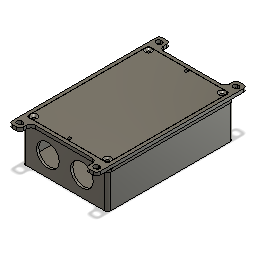
box (Autodesk Fusion 360 design; units mm, degrees)
Autodesk Fusion 360 part; units mm, degrees
sketch "Sketch1" plane through (0, 0, 0) normal (0, 1, 0) x (1, 0, 0)
  line L0 (-39, 48.75) -> (39, 48.75)
  line L1 (39, 48.75) -> (39, -66.25)
  line L2 (39, -66.25) -> (-39, -66.25)
  line L3 (-39, -66.25) -> (-39, 48.75)
  line L4 (0, 70.8126) -> (0, -70.8126) construction
  line L5 (-33.9373, 0) -> (33.9373, 0) construction
  line L6 (-32.25, 35.75) -> (32.25, 35.75) construction
  line L7 (32.25, 35.75) -> (32.25, -35.75) construction
  line L8 (32.25, -35.75) -> (-32.25, -35.75) construction
  line L9 (-32.25, -35.75) -> (-32.25, 35.75) construction
  line L10 (-37, 46.75) -> (37, 46.75)
  line L11 (37, 46.75) -> (37, -64.25)
  line L12 (37, -64.25) -> (-37, -64.25)
  line L13 (-37, -64.25) -> (-37, 46.75)
  circle A0 centre (-32.25, -35.75) radius 3
  circle A1 centre (32.25, -35.75) radius 3
  circle A2 centre (32.25, 35.75) radius 3
  circle A3 centre (-32.25, 35.75) radius 3
  line L14 (-31, 46.75) -> (-31, 43.35)
  line L15 (-33.6, 40.75) -> (-37, 40.75)
  circle A4 centre (-33.6, 43.35) radius 1.3
  arc A5 (-33.6, 40.75) -> (-31, 43.35) centre (-33.6, 43.35) ccw
  line L16 (-33.6, 43.35) -> (-31, 43.35) construction
  line L17 (-33.6, 43.35) -> (-33.6, 40.75) construction
  line L18 (33.6, 40.75) -> (37, 40.75)
  arc A6 (31, 43.35) -> (33.6, 40.75) centre (33.6, 43.35) ccw
  circle A7 centre (33.6, 43.35) radius 1.3
  line L19 (31, 46.75) -> (31, 43.35)
  line L20 (-31, -60.85) -> (-31, -64.25)
  arc A8 (-31, -60.85) -> (-33.6, -58.25) centre (-33.6, -60.85) ccw
  line L21 (-37, -58.25) -> (-33.6, -58.25)
  circle A9 centre (-33.6, -60.85) radius 1.3
  line L22 (-33.6, -60.85) -> (-33.6, -58.25) construction
  line L23 (-33.6, -60.85) -> (-31, -60.85) construction
  line L24 (33.6, -60.85) -> (33.6, -58.25) construction
  line L25 (37, -58.25) -> (33.6, -58.25)
  line L26 (31, -60.85) -> (31, -64.25)
  line L27 (33.6, -60.85) -> (31, -60.85) construction
  arc A10 (33.6, -58.25) -> (31, -60.85) centre (33.6, -60.85) ccw
  circle A11 centre (33.6, -60.85) radius 1.3
  circle A12 centre (0, -61.75) radius 1.35
  circle A13 centre (0, 44.25) radius 1.35
  line L28 (-3, 44.25) -> (-3, 46.75)
  line L29 (3, 44.25) -> (3, 46.75)
  arc A14 (-3, 44.25) -> (3, 44.25) centre (0, 44.25) ccw
  line L30 (-3, -61.75) -> (-3, -64.25)
  line L31 (2.9999, -61.7769) -> (2.9777, -64.25)
  arc A15 (2.9999, -61.7769) -> (-3, -61.75) centre (0, -61.75) ccw
  circle A16 centre (-32.25, 35.75) radius 1.25
  circle A17 centre (32.25, 35.75) radius 1.25
  circle A18 centre (32.25, -35.75) radius 1.25
  circle A19 centre (-32.25, -35.75) radius 1.25
  point P0 (-31, 40.75)
  point P1 (37, -64.25)
  point P2 (37, -64.25)
  dimension "d1" = 78
  dimension "d2" = 115
  dimension "d4" = 71.5
  dimension "d6" = 64.5
  dimension "d7" = 2
  dimension "d8" = 2
  dimension "d9" = 2
  dimension "d10" = 2
  dimension "d11" = 6
  dimension "d12" = 11
  dimension "d31" = 6
  dimension "d32" = 2.6
  dimension "d37" = 2.6
  dimension "d114" = 106
  dimension "d115" = 2.7
  dimension "d116" = 4.5
  dimension "d117" = 3
  dimension "d143" = 2.5
  constraint horizontal L0
  constraint vertical L1
  constraint horizontal L2
  constraint vertical L3
  constraint vertical L4
  constraint midpoint origin L4
  constraint horizontal L5
  constraint midpoint origin L5
  constraint symmetric L1 L3 L4
  constraint horizontal L6
  constraint vertical L7
  constraint horizontal L8
  constraint vertical L9
  constraint symmetric L4 L7 L9
  constraint symmetric L5 L6 L8
  constraint horizontal L10
  constraint vertical L11
  constraint horizontal L12
  constraint vertical L13
  constraint coincident L8.end L9.start
  constraint coincident L7.end L8.start
  constraint coincident L6.end L7.start
  constraint coincident L6.start L9.end
  constraint equal A0 A1
  constraint equal A1 A2
  constraint equal A2 A3
  constraint vertical L14
  constraint horizontal L15
  constraint equal L14 L15
  constraint coincident L10.start L13.end
  constraint coincident L12.end L13.start
  constraint coincident L13 L15.end
  constraint coincident L10 L14.start
  constraint coincident P0 L14
  constraint coincident P0 L15
  constraint tangent L14 A5
  constraint tangent L15 A5
  constraint coincident A4.centre A5.centre
  constraint symmetric L4 L14.start L19.start
  constraint symmetric L4 L15.end L18.end
  constraint symmetric L4 A4 A7
  constraint symmetric L4 L14.end A6.start
  constraint symmetric L4 L15.start L18.start
  constraint symmetric L4 A5 A6
  constraint equal L20 L21
  constraint tangent A8 L21
  constraint tangent L20 A8
  constraint coincident A8.centre A9.centre
  constraint coincident L13 L21.start
  constraint coincident L12 L20.end
  constraint horizontal L21
  constraint vertical L20
  constraint equal L15 L21
  constraint equal A4 A9
  constraint equal A5 A8
  constraint symmetric L4 L12.end P2
  constraint symmetric L4 L21.start L25.start
  constraint symmetric L4 L20.end L26.end
  constraint symmetric L4 A8.end L24.end
  constraint symmetric L4 A8.centre L24.start
  constraint symmetric L4 L20.start L26.start
  constraint symmetric L4 A8 A10
  constraint symmetric L4 A9 A11
  constraint coincident L4 A12.centre
  constraint coincident L4 A13.centre
  constraint equal A12 A13
  constraint concentric A13 A14
  constraint coincident L10 L28.end
  constraint perpendicular L10 L28
  constraint coincident L29.start A14
  constraint coincident L10 L29.end
  constraint perpendicular L10 L29
  constraint coincident L29 A14.end
  constraint tangent L28 A14
  constraint tangent L29 A14
  constraint concentric A12 A15
  constraint coincident L30.start A15
  constraint coincident L12 L30.end
  constraint perpendicular L12 L30
  constraint coincident L12 L31.end
  constraint tangent L31 A15
  constraint coincident L30 A15.end
  constraint tangent L30 A15
  constraint equal A14 A15
  constraint concentric A3 A16
  constraint equal A18 A19
  constraint equal A17 A18
  constraint equal A16 A17
  measures "d1" distance of L0.start L0.end
  measures "d2" distance of L0.start L2.end
  measures "d4" distance of L6 L8
  measures "d6" distance of L7 L9
  measures "d7" distance of L0 L10
  measures "d8" distance of L3 L13
  measures "d9" distance of L1 L11
  measures "d10" distance of L2 L12
  measures "d11" diameter of A0
  measures "d12" distance of L10 L6.start
  measures "d31" distance of P0 L15.end
  measures "d32" diameter of A4
  measures "d37" radius of A5
  measures "d114" distance of A12.centre A13.centre
  measures "d115" diameter of A13
  measures "d116" distance of L0 A13.centre
  measures "d117" radius of A14
  measures "d143" diameter of A16
extrude "Extrude1" add sketch "Sketch1" against normal blind 3 contours L0 L1 L2 L3 | L10 L13 L14 L15 A5 | L10 L11 L12 L13 L14 L15 A5 L18 A6 L19 L20 A8 L21 L25 L26 A10 L28 L29 A14 L30 L31 A15 | L10 L28 L29 A14 | L12 L13 L20 A8 L21 | L10 L11 L18 A6 L19 | L12 L30 L31 A15 | L11 L12 L25 L26 A10 | A0 | A1 | A2 | A3 | A4 | A7 | A9 | A11 | A12 | A13 | A16 | A17 | A18 | A19 makes body 1
extrude "Extrude2" add sketch "Sketch1" along normal blind 31 contours L0 L1 L2 L3 bodies 1
extrude "Extrude9" add sketch "Sketch1" along normal blind 25.8 contours L10 L13 L14 L15 A5 | L12 L13 L20 A8 L21 | L10 L11 L18 A6 L19 | L11 L12 L25 L26 A10 bodies 1
extrude "Extrude3" add sketch "Sketch1" along normal blind 4.5 contours A0 | A1 | A2 | A3 bodies 1
sketch "Sketch11" plane through (0, 31, 0) normal (0, 1, 0) x (1, 0, 0)
  line L0 (-37, 59.75) -> (-33, 59.75)
  line L1 (-30, 56.75) -> (-30, 48.75)
  line L2 (-30, 48.75) -> (-40, 48.75)
  line L3 (-40, 48.75) -> (-40, 56.75)
  line L4 (-39, 48.75) -> (39, 48.75)
  line L5 (-39, -66.25) -> (-39, 48.75)
  line L6 (39, -66.25) -> (-39, -66.25)
  line L7 (39, 48.75) -> (39, -66.25)
  line L8 (-35.65, 52.6) -> (-34.35, 52.6)
  arc A0 (-34.35, 52.6) -> (-34.35, 56.9) centre (-34.35, 54.75) ccw
  line L9 (-34.35, 56.9) -> (-35.65, 56.9)
  arc A1 (-35.65, 56.9) -> (-35.65, 52.6) centre (-35.65, 54.75) ccw
  line L10 (-35.65, 54.75) -> (-34.35, 54.75) construction
  line L11 (-35, 59.2995) -> (-35, 41.7347) construction
  arc A2 (-37, 59.75) -> (-40, 56.75) centre (-37, 56.75) ccw
  arc A3 (-30, 56.75) -> (-33, 59.75) centre (-33, 56.75) ccw
  line L12 (0, 70.8126) -> (0, -70.8126)
  line L13 (40, 48.75) -> (40, 56.75)
  arc A4 (40, 56.75) -> (37, 59.75) centre (37, 56.75) ccw
  line L14 (37, 59.75) -> (33, 59.75)
  arc A5 (33, 59.75) -> (30, 56.75) centre (33, 56.75) ccw
  line L15 (30, 56.75) -> (30, 48.75)
  arc A6 (34.35, 56.9) -> (34.35, 52.6) centre (34.35, 54.75) ccw
  line L16 (35.65, 52.6) -> (34.35, 52.6)
  arc A7 (35.65, 52.6) -> (35.65, 56.9) centre (35.65, 54.75) ccw
  line L17 (34.35, 56.9) -> (35.65, 56.9)
  line L18 (30, 48.75) -> (40, 48.75)
  line L19 (-65.8478, -8.75) -> (59.599, -8.75) construction
  line L20 (-30, -66.25) -> (-40, -66.25)
  line L21 (-40, -66.25) -> (-40, -74.25)
  arc A8 (-40, -74.25) -> (-37, -77.25) centre (-37, -74.25) ccw
  line L22 (-37, -77.25) -> (-33, -77.25)
  arc A9 (-33, -77.25) -> (-30, -74.25) centre (-33, -74.25) ccw
  line L23 (-30, -74.25) -> (-30, -66.25)
  arc A10 (-35.65, -70.1) -> (-35.65, -74.4) centre (-35.65, -72.25) ccw
  line L24 (-34.35, -74.4) -> (-35.65, -74.4)
  arc A11 (-34.35, -74.4) -> (-34.35, -70.1) centre (-34.35, -72.25) ccw
  line L25 (-35.65, -70.1) -> (-34.35, -70.1)
  line L26 (30, -74.25) -> (30, -66.25)
  arc A12 (30, -74.25) -> (33, -77.25) centre (33, -74.25) ccw
  line L27 (37, -77.25) -> (33, -77.25)
  arc A13 (37, -77.25) -> (40, -74.25) centre (37, -74.25) ccw
  line L28 (40, -66.25) -> (40, -74.25)
  arc A14 (35.65, -74.4) -> (35.65, -70.1) centre (35.65, -72.25) ccw
  line L29 (35.65, -70.1) -> (34.35, -70.1)
  arc A15 (34.35, -70.1) -> (34.35, -74.4) centre (34.35, -72.25) ccw
  line L30 (34.35, -74.4) -> (35.65, -74.4)
  line L31 (30, -66.25) -> (40, -66.25)
  line L32 (37, -64.25) -> (-37, -64.25)
  line L33 (-37, -64.25) -> (-37, 46.75)
  line L34 (-37, 46.75) -> (37, 46.75)
  line L35 (37, 46.75) -> (37, -64.25)
  line L36 (-39, -66.25) -> (39, -66.25)
  line L37 (39, -66.25) -> (39, 48.75)
  line L38 (39, 48.75) -> (-39, 48.75)
  line L39 (-39, 48.75) -> (-39, -66.25)
  line L40 (-30, 49.75) -> (30, 49.75)
  line L41 (-30, -67.25) -> (30, -67.25)
  line L42 (-3, 44.25) -> (-3, 46.75)
  arc A16 (-3, 44.25) -> (3, 44.25) centre (0, 44.25) ccw
  circle A17 centre (0, 44.25) radius 1.35
  line L43 (3, 44.25) -> (3, 46.75)
  line L44 (-3, -61.75) -> (-3, -64.25)
  arc A18 (2.9999, -61.7769) -> (-3, -61.75) centre (0, -61.75) ccw
  circle A19 centre (0, -61.75) radius 1.35
  line L45 (2.9999, -61.7769) -> (2.9777, -64.25)
  point P0 (-30, 59.75)
  dimension "d118" = 11
  dimension "d119" = 3
  dimension "d120" = 10
  dimension "d121" = 1.3
  dimension "d122" = 2.15
  dimension "d123" = 5
  dimension "d124" = 40
  dimension "d125" = 127
  dimension "d133" = 1
  constraint horizontal L0
  constraint vertical L1
  constraint horizontal L2
  constraint vertical L3
  constraint tangent L8 A0
  constraint tangent A0 L9
  constraint parallel L8 L9
  constraint tangent L9 A1
  constraint tangent L8 A1
  constraint horizontal L10
  constraint vertical L11
  constraint symmetric A1.centre A0.centre L11
  constraint symmetric L1 L3 L11
  constraint tangent L0 A2
  constraint tangent L3 A2
  constraint coincident P0 L0
  constraint coincident P0 L1
  constraint tangent L0 A3
  constraint tangent L1 A3
  constraint equal A2 A3
  constraint coincident L1.end L4
  constraint symmetric L1.end L12 L15.end
  constraint symmetric L2.end L12 L13.start
  constraint symmetric L8.start L12 L16.start
  constraint symmetric L8.end L12 A6.end
  constraint symmetric A0.end L12 A6.start
  constraint symmetric L9.end L12 A7.end
  constraint symmetric A0 L12 A6
  constraint symmetric A1 L12 A7
  constraint symmetric L0.start L12 A4.end
  constraint symmetric L3.end L12 L13.end
  constraint symmetric A2 L12 A4
  constraint symmetric L0.end L12 L14.end
  constraint symmetric L1.start L12 A5.end
  constraint symmetric A3 L12 A5
  constraint horizontal L19
  constraint symmetric L4 L6 L19
  constraint symmetric L1.end L19 L20.start
  constraint symmetric L2.end L19 L20.end
  constraint symmetric L8.start L19 A10.start
  constraint symmetric L8.end L19 A11.end
  constraint symmetric A0.end L19 L24.start
  constraint symmetric L9.end L19 A10.end
  constraint symmetric A0 L19 A11
  constraint symmetric A1 L19 A10
  constraint symmetric L0.start L19 A8.end
  constraint symmetric L3.end L19 L21.end
  constraint symmetric A2 L19 A8
  constraint symmetric L0.end L19 L22.end
  constraint symmetric L1.start L19 A9.end
  constraint symmetric A3 L19 A9
  constraint symmetric L13.start L19 L28.start
  constraint symmetric L13.end L19 A13.end
  constraint symmetric A4.end L19 L27.start
  constraint symmetric A4 L19 A13
  constraint symmetric L14.end L19 A12.end
  constraint symmetric A5.end L19 L26.start
  constraint symmetric A5 L19 A12
  constraint symmetric L15.end L19 L26.end
  constraint symmetric A6.end L19 L29.end
  constraint symmetric A6.start L19 A15.end
  constraint symmetric A6 L19 A15
  constraint symmetric L16.start L19 A14.end
  constraint symmetric A7.end L19 A14.start
  constraint symmetric A7 L19 A14
  constraint coincident L1 L40.start
  constraint coincident L15 L40.end
  constraint perpendicular L15 L40
  constraint symmetric L19 L40.start L41.start
  constraint symmetric L19 L40.end L41.end
  measures "d118" distance of P0 L1.end
  measures "d119" radius of A2
  measures "d120" distance of L1 L3
  measures "d121" distance of A1.centre A0.centre
  measures "d122" radius of A0
  measures "d123" distance of L0 L10
  measures "d124" distance of L3 L12
  measures "d125" distance of A1.centre A10.centre
  measures "d133" distance of L4 L40
extrude "Extrude19" add sketch "Sketch11" along normal blind 3 contours L0 L1 L2 L3 L4 A2 A3 L38 | L1 L4 L12 L38 L40 | L2 L4 L5 L6 L12 L20 L32 L33 L34 L36 L38 L39 | L4 L12 L15 L38 L40 | L6 L20 L21 A8 L22 A9 L23 L36 | L4 L6 L7 L12 L18 L31 L32 L34 L35 L36 L37 L38 | L4 L13 A4 L14 A5 L15 L18 L38 | L6 L12 L23 L36 L41 | L6 L12 L26 L36 L41 | L6 L26 A12 L27 A13 L28 L31 L36 bodies 1
sketch "Sketch12" plane through (0, 0, 66.25) normal (0, 0, 1) x (1, 0, 0)
  line L0 (-39, 31) -> (-39, -3)
  line L1 (-39, -3) -> (39, -3)
  line L2 (39, -3) -> (39, 31)
  line L3 (39, 31) -> (-39, 31)
  line L4 (-39, 31) -> (-39, -3)
  line L5 (-39, 31) -> (-40, 31)
  line L6 (-40, 31) -> (-39, 27.4807)
  line L7 (0, -6.3909) -> (0, 38.1593) construction
  line L8 (40, 31) -> (39, 27.4807)
  line L9 (39, -3) -> (39, 31)
  line L10 (39, 31) -> (40, 31)
  line L11 (-40, 31) -> (-40, 34)
  line L12 (-39, 34) -> (-40, 34)
  line L13 (-39, 34) -> (-39, 31)
  line L14 (40, 34) -> (39, 34)
  line L15 (40, 31) -> (40, 34)
  line L16 (39, 34) -> (39, 31)
  constraint coincident L5.end L6.start
  constraint coincident L4 L6.end
  constraint symmetric L5.end L7 L8.start
  constraint symmetric L6.end L7 L8.end
  constraint coincident L12.start L13.start
  constraint coincident L0.start L3.end
  constraint coincident L14.end L16.start
  constraint coincident L2.end L3.start
  constraint coincident L8.start L10.end
extrude "Extrude20" add sketch "Sketch12" against normal blind 115 contours L0 L4 L5 L6 | L5 L11 L12 L13 | L2 L8 L9 L10 | L10 L14 L15 L16 bodies 1
sketch "Sketch13" plane through (39, 0, 0) normal (1, 0, 0) x (0, 0, -1)
  line L0 (48.75, 27.4807) -> (-66.25, 27.4807)
  line L1 (-66.25, 27.4807) -> (-66.25, -3)
  line L2 (-66.25, -3) -> (48.75, -3)
  line L3 (48.75, -3) -> (48.75, 27.4807)
  line L4 (-74.25, 31) -> (-67.25, 31)
  line L5 (48.75, 27.4807) -> (-66.25, 27.4807)
  line L6 (-66.25, 27.4807) -> (-67.25, 31)
  line L7 (-66.25, 31) -> (-74.25, 31)
  line L8 (-66.25, 31) -> (-66.25, 27.4807)
  line L9 (48.75, 31) -> (48.75, 27.4807)
  line L10 (48.75, 31) -> (56.75, 31)
  line L11 (48.75, 27.4807) -> (49.75, 31)
  point P0 (49.75, 31)
  constraint coincident L0.end L1.start
  constraint coincident L4.end L6.end
  constraint coincident L0.start L3.end
  constraint coincident P0 L11.end
sketch "Sketch3" plane through (0, 0, 66.25) normal (0, 0, 1) x (1, 0, 0)
  line L0 (-39, 27.4807) -> (-39, -3)
  line L1 (-39, -3) -> (39, -3)
  line L2 (39, -3) -> (39, 27.4807)
  line L3 (-47.6464, 15) -> (51.1044, 15) construction
  circle A0 centre (-15.5, 15) radius 10.25
  circle A1 centre (15.5, 15) radius 10.25
  line L4 (0, 0) -> (0, 33.0794) construction
  circle A2 centre (15.5, 15) radius 15
  circle A3 centre (-15.5, 15) radius 15
  line L5 (-40, 31) -> (-39, 27.4807)
  line L6 (39, 27.4807) -> (40, 31)
  line L7 (40, 31) -> (-40, 31)
  dimension "d22" = 33
  dimension "d24" = 31
  dimension "d25" = 20.5
  dimension "d41" = 15
  dimension "d55" = 30
  constraint horizontal L3
  constraint coincident L3 A0.centre
  constraint coincident L3 A1.centre
  constraint equal A0 A1
  constraint coincident L4.start origin
  constraint perpendicular L3 L4
  constraint symmetric A0 A1 L4
  constraint concentric A1 A2
  constraint concentric A0 A3
  constraint equal A2 A3
  measures "d24" distance of A0.centre A1.centre
  measures "d25" diameter of A0
  measures "d41" distance of L4.start L3
  measures "d55" diameter of A3
extrude "Extrude5" cut sketch "Sketch3" against normal blind 3 contours A0 | A1 bodies 1
fillet "Fillet1" radius 3 8 edges at (-39, 12.2404, -48.75) (-39, 12.2404, 66.25) (39, 12.2404, -48.75) (39, 12.2404, 66.25) (39.5, 29.2404, 66.25) (39.5, 29.2404, -48.75) (-39.5, 29.2404, -48.75) (-39.5, 29.2404, 66.25) on bodies 1
fillet "Fillet1" radius 2 4 edges at (37, 29.9, -46.75) (37, 29.9, 64.25) (-37, 29.9, 64.25) (-37, 29.9, -46.75) on bodies 1
fillet "Fillet1" radius 4 4 edges at (-30, 32.5, 67.25) (30, 32.5, 67.25) (30, 32.5, -49.75) (-30, 32.5, -49.75) on bodies 1
sketch "Sketch14" plane through (0, 34, 0) normal (0, 1, 0) x (-1, 0, 0)
  line L0 (-35.65, 74.4) -> (-34.35, 74.4)
  arc A0 (-34.35, 70.1) -> (-34.35, 74.4) centre (-34.35, 72.25) ccw
  line L1 (-34.35, 70.1) -> (-35.65, 70.1)
  arc A1 (-35.65, 74.4) -> (-35.65, 70.1) centre (-35.65, 72.25) ccw
  arc A2 (34.35, 74.4) -> (34.35, 70.1) centre (34.35, 72.25) ccw
  line L2 (34.35, 74.4) -> (35.65, 74.4)
  arc A3 (35.65, 70.1) -> (35.65, 74.4) centre (35.65, 72.25) ccw
  line L3 (35.65, 70.1) -> (34.35, 70.1)
  arc A4 (35.65, -56.9) -> (35.65, -52.6) centre (35.65, -54.75) ccw
  line L4 (35.65, -56.9) -> (34.35, -56.9)
  arc A5 (34.35, -52.6) -> (34.35, -56.9) centre (34.35, -54.75) ccw
  line L5 (34.35, -52.6) -> (35.65, -52.6)
  line L6 (35, -46.75) -> (-35, -46.75)
  line L7 (-37, -44.75) -> (-37, 62.25)
  line L8 (-35, 64.25) -> (35, 64.25)
  line L9 (37, 62.25) -> (37, -44.75)
  arc A6 (-35.65, -52.6) -> (-35.65, -56.9) centre (-35.65, -54.75) ccw
  line L10 (-35.65, -52.6) -> (-34.35, -52.6)
  arc A7 (-34.35, -56.9) -> (-34.35, -52.6) centre (-34.35, -54.75) ccw
  line L11 (-34.35, -56.9) -> (-35.65, -56.9)
  line L12 (40, -56.75) -> (40, 74.25)
  arc A8 (40, 74.25) -> (37, 77.25) centre (37, 74.25) ccw
  line L13 (37, 77.25) -> (33, 77.25)
  arc A9 (33, 77.25) -> (30, 74.25) centre (33, 74.25) ccw
  line L14 (30, 74.25) -> (30, 71.25)
  line L15 (26, 67.25) -> (-26, 67.25)
  line L16 (-30, 71.25) -> (-30, 74.25)
  arc A10 (-30, 74.25) -> (-33, 77.25) centre (-33, 74.25) ccw
  line L17 (-33, 77.25) -> (-37, 77.25)
  arc A11 (-37, 77.25) -> (-40, 74.25) centre (-37, 74.25) ccw
  line L18 (-40, 74.25) -> (-40, -56.75)
  arc A12 (-40, -56.75) -> (-37, -59.75) centre (-37, -56.75) ccw
  line L19 (-37, -59.75) -> (-33, -59.75)
  arc A13 (-33, -59.75) -> (-30, -56.75) centre (-33, -56.75) ccw
  line L20 (-30, -56.75) -> (-30, -53.75)
  line L21 (-26, -49.75) -> (26, -49.75)
  line L22 (30, -53.75) -> (30, -56.75)
  arc A14 (30, -56.75) -> (33, -59.75) centre (33, -56.75) ccw
  line L23 (33, -59.75) -> (37, -59.75)
  arc A15 (37, -59.75) -> (40, -56.75) centre (37, -56.75) ccw
  line L24 (34.8, -44.55) -> (-34.8, -44.55)
  line L25 (34.8, 62.05) -> (34.8, -44.55)
  line L26 (-34.8, 62.05) -> (34.8, 62.05)
  line L27 (-34.8, -44.55) -> (-34.8, 62.05)
  arc A16 (-36.8, -44.75) -> (-35, -46.55) centre (-35, -44.75) ccw
  line L28 (35, -46.55) -> (-35, -46.55)
  arc A17 (35, -46.55) -> (36.8, -44.75) centre (35, -44.75) ccw
  line L29 (36.8, 62.25) -> (36.8, -44.75)
  arc A18 (36.8, 62.25) -> (35, 64.05) centre (35, 62.25) ccw
  line L30 (-35, 64.05) -> (35, 64.05)
  arc A19 (-35, 64.05) -> (-36.8, 62.25) centre (-35, 62.25) ccw
  line L31 (-36.8, -44.75) -> (-36.8, 62.25)
  line L32 (33.6, 58.25) -> (37, 58.25)
  arc A20 (31, 60.85) -> (33.6, 58.25) centre (33.6, 60.85) ccw
  line L33 (31, 64.25) -> (31, 60.85)
  line L34 (-31, 60.85) -> (-31, 64.25)
  arc A21 (-33.6, 58.25) -> (-31, 60.85) centre (-33.6, 60.85) ccw
  line L35 (-37, 58.25) -> (-33.6, 58.25)
  line L36 (-33.6, -40.75) -> (-37, -40.75)
  arc A22 (-31, -43.35) -> (-33.6, -40.75) centre (-33.6, -43.35) ccw
  line L37 (-31, -46.75) -> (-31, -43.35)
  line L38 (37, -40.75) -> (33.6, -40.75)
  arc A23 (33.6, -40.75) -> (31, -43.35) centre (33.6, -43.35) ccw
  line L39 (31, -43.35) -> (31, -46.75)
  line L40 (0, 72.7504) -> (0, -56.2733) construction
  circle A24 centre (0, -44.25) radius 1.35
  circle A25 centre (0, 61.75) radius 1.35
  line L41 (14.313, 8.75) -> (-20.1597, 8.75) construction
  line L42 (-26, -49.75) -> (26, -49.75)
  line L43 (26, 67.25) -> (-26, 67.25)
  circle A26 centre (0, -44.25) radius 3
  circle A27 centre (0, 61.75) radius 3
  circle A28 centre (33.6, -43.35) radius 1.5
  circle A29 centre (-33.6, -43.35) radius 1.5
  circle A30 centre (-33.6, 60.85) radius 1.5
  circle A31 centre (33.6, 60.85) radius 1.5
  arc A32 (-37, -44.75) -> (-35, -46.75) centre (-35, -44.75) ccw
  arc A33 (-35, 64.25) -> (-37, 62.25) centre (-35, 62.25) ccw
  arc A34 (37, 62.25) -> (35, 64.25) centre (35, 62.25) ccw
  arc A35 (35, -46.75) -> (37, -44.75) centre (35, -44.75) ccw
  arc A36 (26, 67.25) -> (30, 71.25) centre (26, 71.25) ccw
  arc A37 (-30, 71.25) -> (-26, 67.25) centre (-26, 71.25) ccw
  arc A38 (-26, -49.75) -> (-30, -53.75) centre (-26, -53.75) ccw
  arc A39 (30, -53.75) -> (26, -49.75) centre (26, -53.75) ccw
  dimension "d150" = 106
  dimension "d151" = 2.7
  dimension "d152" = 6
  dimension "d157" = 3
  constraint vertical L40
  constraint coincident origin L40
  constraint coincident L40 A24.centre
  constraint coincident L40 A25.centre
  constraint equal A24 A25
  constraint horizontal L41
  constraint symmetric L41 L42 L43
  constraint symmetric A24 A25 L41
  constraint concentric A24 A26
  constraint concentric A25 A27
  constraint equal A26 A27
  constraint concentric A23 A28
  constraint concentric A22 A29
  constraint concentric A21 A30
  constraint concentric A20 A31
  constraint equal A30 A31
  constraint equal A29 A30
  constraint equal A28 A29
  constraint parallel L6 L24
  constraint parallel L9 L25
  constraint parallel L8 L26
  constraint parallel L7 L27
  constraint parallel L6 L28
  constraint parallel L9 L29
  constraint parallel L8 L30
  constraint parallel L7 L31
  constraint tangent A19 L31
  constraint tangent L30 A19
  constraint tangent A18 L30
  constraint tangent L29 A18
  constraint tangent A17 L29
  constraint tangent L28 A17
  constraint tangent A16 L28
  constraint tangent A16 L31
  measures "d150" distance of A24.centre A25.centre
  measures "d151" diameter of A24
  measures "d152" diameter of A26
  measures "d157" diameter of A28
extrude "Extrude24" add sketch "Sketch14" against normal blind 2 separate body contours L24 L25 L28 A17 L29 L38 L39 A28 | L24 L28 L39 A26 | L24 L28 A24 A26 | L24 L25 L38 A23 L39 A28 | L24 L25 L26 L27 L32 A20 L33 L34 A21 L35 L36 A22 L37 L38 A23 L39 A26 A27 | L25 L29 L32 L38 | L24 L28 L37 A26 | L24 A24 A26 | L25 L26 L29 A18 L30 L32 L33 A31 | L24 L27 A16 L28 L31 L36 L37 A29 | L24 L25 A28 | L25 L26 L32 A20 L33 A31 | L24 L27 L36 A22 L37 A29 | L26 L30 L33 A27 | L25 L26 A31 | L27 L31 L35 L36 | L24 L27 A29 | L26 L30 A25 A27 | L26 L27 L30 A19 L31 L34 L35 A30 | L26 L30 L34 A27 | L26 A25 A27 | L26 L27 L34 A21 L35 A30 | L26 L27 A30 picked at (34.7063, -44.4563) picked at (34.7063, 61.9563) picked at (-34.7063, -44.4563) picked at (-34.7063, 61.9563) makes body 2
extrude "Extrude25" add sketch "Sketch14" against normal blind 8 contours L24 L25 L28 A17 L29 L38 L39 A28 | L24 L28 L39 A26 | L24 L28 A24 A26 | L24 L25 L38 A23 L39 A28 | L25 L29 L32 L38 | L24 L28 L37 A26 | L24 A24 A26 | L25 L26 L29 A18 L30 L32 L33 A31 | L24 L27 A16 L28 L31 L36 L37 A29 | L24 A24 | L24 A24 | L24 L25 A28 | L25 L26 L32 A20 L33 A31 | L24 L27 L36 A22 L37 A29 | L26 L30 L33 A27 | L25 L26 A31 | L27 L31 L35 L36 | L24 L27 A29 | L26 L30 A25 A27 | L26 L27 L30 A19 L31 L34 L35 A30 | L26 L30 L34 A27 | L26 A25 A27 | L26 L27 L34 A21 L35 A30 | L26 A25 | L26 A25 | L26 L27 A30 picked at (34.7063, -44.4563) picked at (34.7063, 61.9563) picked at (-34.7063, -44.4563) picked at (-34.7063, 61.9563) bodies 2
extrude "Extrude26" cut sketch "Sketch14" against normal blind 7 contours L24 A24 | L24 A24 | L26 A25 | L26 A25 bodies 2
extrude "Extrude27" cut sketch "Sketch3" against normal blind 15 contours A2 | A3 bodies 2
chamfer "Chamfer5" distance 1.6 angle 45 4 edges at (-32.2015, 34, -42.8076) (34.9985, 34, -42.8076) (34.9985, 34, 61.3924) (-32.2015, 34, 61.3924) on bodies 2
equation "d6 = 67.5 mm - 3 mm"
equation "d116 = ( d2 - d114 ) / 2"
named bodies: "Body", "Cover"
